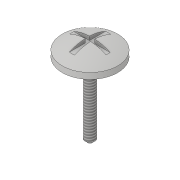
# Autodesk Inventor part: 零件3
Saved by Autodesk Inventor 2019 (Build 230136000, 136)
## iProperties
Created: 2022-10-02
Part Number: 零件3
Material: Generic
Document SubType Name: Modeling
Designer: user
Density: 1 g/cm^3
Appearance: Default
Author: user
Autodesk Inventor part; units mm, degrees
ref_plane "YZ Plane" through (0, 0, 0) normal (1, 0, 0) x (0, 1, 0)
ref_plane "XZ Plane" through (0, 0, 0) normal (0, 1, 0) x (-1, 0, 0)
sketch "草圖1" plane through (0, 0, 0) normal (0, 0, 1) x (1, 0, 0)
  arc A0 (1.4, 0.0728) -> (0, 0.5675) centre (0, -1.6606) ccw
  line L0 (0, 1.1572) -> (0, -2.1303) projected
  line L1 (0, 0.0728) -> (0, 0.5675)
  line L2 (0, 0.0728) -> (1.4, 0.0728)
  dimension "d11" = 1.4
  constraints: 4 end point, 2 point on circle, 2 point on line, 1 centre point, 1 horizontal
  measures "d11" distance of L1.start L2.end
revolve "迴轉1" add sketch "草圖1" angle 360 about axis through (0, 0, 0) along (0, -1, 0)
ref_plane "工作平面1" through (0, 0.5675, 0) normal (0, -1, 0) x (1, 0, 0)
sketch "草圖2" plane through (0, 0.5675, 0) normal (0, -1, 0) x (1, 0, 0)
  line L0 (-2.9128, 0.1062) -> (2.9128, 0.1062)
  line L1 (2.9128, 0.1062) -> (2.9128, -0.1062)
  line L2 (2.9128, -0.1062) -> (-2.9128, -0.1062)
  line L3 (-2.9128, -0.1062) -> (-2.9128, 0.1062)
  line L4 (-2.9128, 0.1062) -> (2.9128, -0.1062) construction
  line L5 (2.9128, 0.1062) -> (-2.9128, -0.1062) construction
  line L6 (-0.1315, 2.5627) -> (0.1315, 2.5627)
  line L7 (0.1315, 2.5627) -> (0.1315, -2.5627)
  line L8 (0.1315, -2.5627) -> (-0.1315, -2.5627)
  line L9 (-0.1315, -2.5627) -> (-0.1315, 2.5627)
  line L10 (-0.1315, 2.5627) -> (0.1315, -2.5627) construction
  line L11 (0.1315, 2.5627) -> (-0.1315, -2.5627) construction
  point P0 (0, 0)
  constraints: 24 end point, 4 midpoint, 4 parallel, 2 horizontal, 2 perpendicular
extrude "擠出1" cut sketch "草圖2" along normal blind 0.2
sketch "草圖3" plane through (0, 0.0728, 0) normal (0, -1, 0) x (1, 0, 0)
  circle A0 centre (0, 0) radius 0.25
  dimension "d10" = 0.5
  constraints: 1 centre point, 1 coincident
  measures "d10" diameter of A0
extrude "擠出2" add sketch "草圖3" along normal blind 4
chamfer "倒角1" distance 0.125 angle 45 1 edges at (-0.25, -3.9272, 0)
sketch "草圖4" plane through (0, 0.0728, 0) normal (0, -1, 0) x (1, 0, 0)
  circle A0 centre (0, 0) radius 0.25 projected
  circle A1 centre (0, 0) radius 1.4 projected
extrude "擠出3" add sketch "草圖4" along normal blind 0.3 contours A0 | A1
thread "螺紋2" size "M0.5x0.125" class "6g" standard "ANSI Metric M Profile" full length
